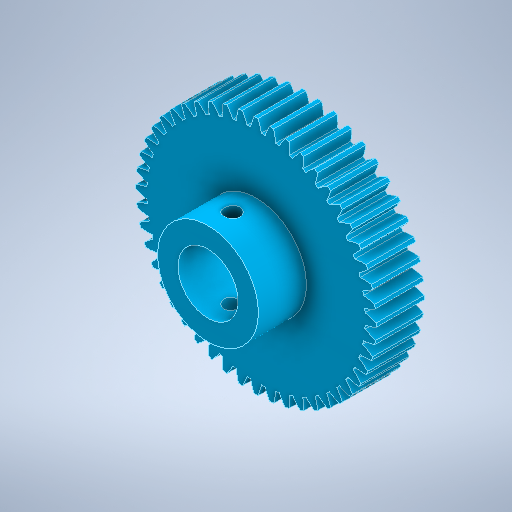
# Autodesk Inventor part: 平歯車1
Saved by Autodesk Inventor 2025.1 (Build 291241000, 241)
## iProperties
CustomPartVersion: 1
Created: 2024-10-03
Part Number: 平歯車1
Material: Steel
Document SubType Name: Modeling
Designer: yuki0520
Categories: <?xml version="1.0" encoding="UTF-16"?> <MemberInstance><Categories><FamilyTemplate><FamilyTemplateParameter ValueType="xs:double" Id="1" ObjectReferenceKey="da_z" ObjectType="kUserParameterObject"/><FamilyTemplateParameter ValueType="xs:double" Id="2" ObjectReferenceKey="da_b" ObjectType="kUserParameterObject"/><FamilyTemplateParameter ValueType="xs:double" Id="3" ObjectReferenceKey="da_beta" ObjectType="kUserParameterObject"/><FamilyTemplateParameter ValueType="xs:double" Id="4" ObjectReferenceKey="da_da" ObjectType="kUserParameterObject"/><FamilyTemplateParameter ValueType="xs:double" Id="5" ObjectReferenceKey="da_aw" ObjectType="kUserParameterObject"/><FamilyTemplateParameter ValueType="xs:string" Id="6" ObjectReferenceKey="EAIAABAAAACIAQAAAAAAAIAAAAAAAAAA" ObjectType="83910656" SubObjectId="SurfaceGeometry"/></FamilyTemplate><ParamToTemplateMap><ParamToTemplate CategoryParameter="//CategoryParameter[@InternalName='046C89C9-8512-4d59-83FE-43B91F4F132A']" TemplateParameter="1"/><ParamToTemplate CategoryParameter="//CategoryParameter[@InternalName='2552DF32-E462-4b46-AEBF-C6C7768E72AC']" TemplateParameter="2"/><ParamToTemplate CategoryParameter="//CategoryParameter[@InternalName='C9EE641D-15FC-4fae-A226-E94C4372FDD7']" TemplateParameter="3"/><ParamToTemplate><ParamToTemplate CategoryParameter="//CategoryParameter[@InternalName='00B6519A-459B-49c7-AD84-2E56D39A5744']" ConstantValue="0.000000"/></ParamToTemplate><ParamToTemplate><ParamToTemplate CategoryParameter="//CategoryParameter[@InternalName='04B31F0E-C7A6-4894-AA32-9629BEFACF47']" ConstantValue="1.000000"/></ParamToTemplate><ParamToTemplate><ParamToTemplate CategoryParameter="//CategoryParameter[@InternalName='43CBEC2E-7847-49e7-A936-2F7889FCB2D9']" ConstantValue="0.250000"/></ParamToTemplate><ParamToTemplate><ParamToTemplate CategoryParameter="//CategoryParameter[@InternalName='B1EFC894-105D-4ebd-86BF-FA20ED196853']" ConstantValue="0.350000"/></ParamToTemplate><ParamToTemplate><ParamToTemplate CategoryParameter="//CategoryParameter[@InternalName='51175063-3D10-4879-93E8-6246FE8B403D']" ConstantValue="2060000000.000000"/></ParamToTemplate><ParamToTemplate><ParamToTemplate CategoryParameter="//CategoryParameter[@InternalName='A3A52E27-4454-46a9-B0BD-C932399B70AF']" ConstantValue="0.300000"/></ParamToTemplate><ParamToTemplate><ParamToTemplate CategoryParameter="//CategoryParameter[@InternalName='91B76062-C214-41d9-B1B9-14D2AB99603D']" ConstantValue="0.100000"/></ParamToTemplate><ParamToTemplate><ParamToTemplate CategoryParameter="//CategoryParameter[@InternalName='374E806E-8B8A-4dda-A9AA-1039D6500AD2']" ConstantValue="10.000000"/></ParamToTemplate><ParamToTemplate><ParamToTemplate CategoryParameter="//CategoryParameter[@InternalName='2D373A89-B862-43d6-8D0B-0CBF12AB9F6C']" ConstantValue="0.349066"/></ParamToTemplate><ParamToTemplate CategoryParameter="//CategoryParameter[@InternalName='37777632-D6A2-4fac-9D53-DB8ACD95C989']" TemplateParameter="4"/><ParamToTemplate CategoryParameter="//CategoryParameter[@InternalName='FD1017F1-B727-4f7e-9707-0F86F1FF9423']" TemplateParameter="5"/><ParamToTemplate><ParamToTemplate CategoryParameter="//CategoryParameter[@InternalName='9E1B4470-B2D3-4ff1-B813-535BB4CDF51A']" ConstantValue="3520000.000000"/></ParamToTemplate><ParamToTemplate><ParamToTemplate CategoryParameter="//CategoryParameter[@InternalName='F8452263-BFF6-458c-9FB1-07C4B99E95CD']" ConstantValue="11400000.000000"/></ParamToTemplate><ParamToTemplate><ParamToTemplate CategoryParameter="//CategoryParameter[@InternalName='3E3BB259-FD49-497f-8171-6EBC954A3479']" ConstantValue="2.000000"/></ParamToTemplate><ParamToTemplate CategoryParameter="//CategoryParameter[@InternalName='27C3BAF2-7550-4e4b-AE2C-0DB134B7D9B7']" TemplateParameter="6"/></ParamToTemplateMap><Category DisplayName="Gear" InternalName="DC85795E-93AB-48d5-8EEE-5A27447B64BD" Mnemonic="Gear"><CategoryParameter DisplayName="z" InternalName="046C89C9-8512-4d59-83FE-43B91F4F132A" Mnemonic="z"/><CategoryParameter DisplayName="b" InternalName="2552DF32-E462-4b46-AEBF-C6C7768E72AC" Mnemonic="b"/><CategoryParameter DisplayName="||b|" InternalName="C9EE641D-15FC-4fae-A226-E94C4372FDD7" Mnemonic="beta"/><CategoryParameter DisplayName="x" InternalName="00B6519A-459B-49c7-AD84-2E56D39A5744" Mnemonic="x"/><CategoryParameter DisplayName="a*" InternalName="04B31F0E-C7A6-4894-AA32-9629BEFACF47" Mnemonic="a"/><CategoryParameter DisplayName="c*" InternalName="43CBEC2E-7847-49e7-A936-2F7889FCB2D9" Mnemonic="c"/><CategoryParameter DisplayName="r|.f|*" InternalName="B1EFC894-105D-4ebd-86BF-FA20ED196853" Mnemonic="rf"/><CategoryParameter DisplayName="E" InternalName="51175063-3D10-4879-93E8-6246FE8B403D" Mnemonic="E"/><CategoryParameter DisplayName="||m|" InternalName="A3A52E27-4454-46a9-B0BD-C932399B70AF" Mnemonic="mi"/><Category DisplayName="SpurGear" InternalName="26C5A22E-A91E-4dfd-A3B3-23CCAFAE1764" Mnemonic="SpurGear"><CategoryParameter DisplayName="m" InternalName="91B76062-C214-41d9-B1B9-14D2AB99603D" Mnemonic="m"/><CategoryParameter DisplayName="P" InternalName="374E806E-8B8A-4dda-A9AA-1039D6500AD2" Mnemonic="PP"/><CategoryParameter DisplayName="||a|" InternalName="2D373A89-B862-43d6-8D0B-0CBF12AB9F6C" Mnemonic="alpha"/><CategoryParameter DisplayName="d|.a|" InternalName="37777632-D6A2-4fac-9D53-DB8ACD95C989" Mnemonic="da"/><CategoryParameter DisplayName="a|.w|" InternalName="FD1017F1-B727-4f7e-9707-0F86F1FF9423" Mnemonic="aw"/><CategoryParameter DisplayName="||s||.Flim|" InternalName="9E1B4470-B2D3-4ff1-B813-535BB4CDF51A" Mnemonic="sFlim"/><CategoryParameter DisplayName="||s||.Hlim|" InternalName="F8452263-BFF6-458c-9FB1-07C4B99E95CD" Mnemonic="sHlim"/><CategoryParameter DisplayName="タイプ" InternalName="3E3BB259-FD49-497f-8171-6EBC954A3479" Mnemonic="type"/><CategoryParameter DisplayName="PitchDiameter" InternalName="27C3BAF2-7550-4e4b-AE2C-0DB134B7D9B7" Mnemonic="IDS_PITCHDIAM"/></Category></Category></Categories></MemberInstance>
Density: 1 g/cm^3
Appearance: スカイ ブルー 標準
Author: yuki0520
Autodesk Inventor part; units mm, degrees
sketch "Sketch1" plane through (0, 0, 0) normal (0, 0, 1) x (1, 0, 0)
  circle A0 centre (0, 0) radius 25
  dimension "d0" = 50
  constraints: 1 centre point
  measures "d0" diameter of A0
extrude "Extrusion1" add sketch "Sketch1" along normal blind 10
ref_plane "Work Plane2" through (0, 0, 5) normal (0, 0, 1) x (1, 0, 0)
sketch "Sketch2" plane through (0, 0, 0) normal (0, 0, -1) x (-1, 0, 0)
  circle A0 centre (0, 0) radius 25 projected
  circle A1 centre (0, 0) radius 24
  dimension "d3" = 48
  constraints: 1 centre point, 1 coincident
  measures "d3" diameter of A1
surface extrude "ピッチ円直径" sketch "Sketch2" against normal through all shown no curves A1
ref_plane "Work Plane8" through (0, 0, 0) normal (0.9978589, 0.0654031, 0) x (0, 0, 1)
ref_plane "Work Plane9" through (0, 0, 0) normal (1, 0, 0) x (0, 1, 0)
spur gear teeth "平歯車" teeth 48 pitch diameter 48 tip diameter 50 root diameter 45.5 face width 10 start plane through (0, 0, 0) normal (0, 0, -1) x (-1, 0, 0)
sketch "スケッチ3" plane through (0, 0, 10) normal (0, 0, 1) x (1, 0, 0)
  arc A0 (3.6683, -24.7294) -> (4.0726, -22.3825) centre (-7.7435, -21.5549) ccw projected
  arc A1 (4.0726, -22.3825) -> (4.8028, -22.2373) centre (0, 0) ccw projected
  arc A2 (4.8028, -22.2373) -> (6.0745, -24.2508) centre (15.4028, -16.9508) ccw projected
  arc A3 (6.0745, -24.2508) -> (6.8647, -24.039) centre (0, 0) ccw projected
  arc A4 (6.8647, -24.039) -> (6.9593, -21.6594) centre (-4.8638, -22.3812) ccw projected
  arc A5 (6.9593, -21.6594) -> (7.6642, -21.4201) centre (0, 0) ccw projected
  arc A6 (7.6642, -21.4201) -> (9.1879, -23.2504) centre (17.4835, -14.7953) ccw projected
  arc A7 (9.1879, -23.2504) -> (9.9437, -22.9374) centre (0, 0) ccw projected
  arc A8 (9.9437, -22.9374) -> (9.7269, -20.5658) centre (-1.9009, -22.8246) ccw projected
  arc A9 (9.7269, -20.5658) -> (10.3946, -20.2365) centre (0, 0) ccw projected
  arc A10 (10.3946, -20.2365) -> (12.1441, -21.8523) centre (19.2651, -12.3867) ccw projected
  arc A11 (12.1441, -21.8523) -> (12.8526, -21.4432) centre (0, 0) ccw projected
  arc A12 (12.8526, -21.4432) -> (12.328, -19.1202) centre (1.0946, -22.8774) ccw projected
  arc A13 (12.328, -19.1202) -> (12.947, -18.7066) centre (0, 0) ccw projected
  arc A14 (12.947, -18.7066) -> (14.8925, -20.0802) centre (20.7171, -9.7661) ccw projected
  arc A15 (14.8925, -20.0802) -> (15.5415, -19.5822) centre (0, 0) ccw projected
  arc A16 (15.5415, -19.5822) -> (14.7183, -17.3475) centre (4.0714, -22.5388) ccw projected
  arc A17 (14.7183, -17.3475) -> (15.278, -16.8566) centre (0, 0) ccw projected
  arc A18 (15.278, -16.8566) -> (17.3861, -17.9645) centre (21.8146, -6.9784) ccw projected
  arc A19 (17.3861, -17.9645) -> (17.9645, -17.3861) centre (0, 0) ccw projected
  arc A20 (17.9645, -17.3861) -> (16.8566, -15.278) centre (6.9784, -21.8146) ccw projected
  arc A21 (16.8566, -15.278) -> (17.3475, -14.7183) centre (0, 0) ccw projected
  arc A22 (17.3475, -14.7183) -> (19.5822, -15.5415) centre (22.5388, -4.0714) ccw projected
  arc A23 (19.5822, -15.5415) -> (20.0802, -14.8925) centre (0, 0) ccw projected
  arc A24 (20.0802, -14.8925) -> (18.7066, -12.947) centre (9.7661, -20.7171) ccw projected
  arc A25 (18.7066, -12.947) -> (19.1202, -12.328) centre (0, 0) ccw projected
  arc A26 (19.1202, -12.328) -> (21.4432, -12.8526) centre (22.8774, -1.0946) ccw projected
  arc A27 (21.4432, -12.8526) -> (21.8523, -12.1441) centre (0, 0) ccw projected
  arc A28 (21.8523, -12.1441) -> (20.2365, -10.3946) centre (12.3867, -19.2651) ccw projected
  arc A29 (20.2365, -10.3946) -> (20.5658, -9.7269) centre (0, 0) ccw projected
  arc A30 (20.5658, -9.7269) -> (22.9374, -9.9437) centre (22.8246, 1.9009) ccw projected
  arc A31 (22.9374, -9.9437) -> (23.2504, -9.1879) centre (0, 0) ccw projected
  arc A32 (23.2504, -9.1879) -> (21.4201, -7.6642) centre (14.7953, -17.4835) ccw projected
  arc A33 (21.4201, -7.6642) -> (21.6594, -6.9593) centre (0, 0) ccw projected
  arc A34 (21.6594, -6.9593) -> (24.039, -6.8647) centre (22.3812, 4.8638) ccw projected
  arc A35 (24.039, -6.8647) -> (24.2508, -6.0745) centre (0, 0) ccw projected
  arc A36 (24.2508, -6.0745) -> (22.2373, -4.8028) centre (16.9508, -15.4028) ccw projected
  arc A37 (22.2373, -4.8028) -> (22.3825, -4.0726) centre (0, 0) ccw projected
  arc A38 (22.3825, -4.0726) -> (24.7294, -3.6683) centre (21.5549, 7.7435) ccw projected
  arc A39 (24.7294, -3.6683) -> (24.8362, -2.8572) centre (0, 0) ccw projected
  arc A40 (24.8362, -2.8572) -> (22.6739, -1.8592) centre (18.8162, -13.0585) ccw projected
  arc A41 (22.6739, -1.8592) -> (22.7226, -1.1163) centre (0, 0) ccw projected
  arc A42 (22.7226, -1.1163) -> (24.9967, -0.409) centre (20.3597, 10.4907) ccw projected
  arc A43 (24.9967, -0.409) -> (24.9967, 0.409) centre (0, 0) ccw projected
  arc A44 (24.9967, 0.409) -> (22.7226, 1.1163) centre (20.3597, -10.4907) ccw projected
  arc A45 (22.7226, 1.1163) -> (22.6739, 1.8592) centre (0, 0) ccw projected
  arc A46 (22.6739, 1.8592) -> (24.8362, 2.8572) centre (18.8162, 13.0585) ccw projected
  arc A47 (24.8362, 2.8572) -> (24.7294, 3.6683) centre (0, 0) ccw projected
  arc A48 (24.7294, 3.6683) -> (22.3825, 4.0726) centre (21.5549, -7.7435) ccw projected
  arc A49 (22.3825, 4.0726) -> (22.2373, 4.8028) centre (0, 0) ccw projected
  arc A50 (22.2373, 4.8028) -> (24.2508, 6.0745) centre (16.9508, 15.4028) ccw projected
  arc A51 (24.2508, 6.0745) -> (24.039, 6.8647) centre (0, 0) ccw projected
  arc A52 (24.039, 6.8647) -> (21.6594, 6.9593) centre (22.3812, -4.8638) ccw projected
  arc A53 (21.6594, 6.9593) -> (21.4201, 7.6642) centre (0, 0) ccw projected
  arc A54 (21.4201, 7.6642) -> (23.2504, 9.1879) centre (14.7953, 17.4835) ccw projected
  arc A55 (23.2504, 9.1879) -> (22.9374, 9.9437) centre (0, 0) ccw projected
  arc A56 (22.9374, 9.9437) -> (20.5658, 9.7269) centre (22.8246, -1.9009) ccw projected
  arc A57 (20.5658, 9.7269) -> (20.2365, 10.3946) centre (0, 0) ccw projected
  arc A58 (20.2365, 10.3946) -> (21.8523, 12.1441) centre (12.3867, 19.2651) ccw projected
  arc A59 (21.8523, 12.1441) -> (21.4432, 12.8526) centre (0, 0) ccw projected
  arc A60 (21.4432, 12.8526) -> (19.1202, 12.328) centre (22.8774, 1.0946) ccw projected
  arc A61 (19.1202, 12.328) -> (18.7066, 12.947) centre (0, 0) ccw projected
  arc A62 (18.7066, 12.947) -> (20.0802, 14.8925) centre (9.7661, 20.7171) ccw projected
  arc A63 (20.0802, 14.8925) -> (19.5822, 15.5415) centre (0, 0) ccw projected
  arc A64 (19.5822, 15.5415) -> (17.3475, 14.7183) centre (22.5388, 4.0714) ccw projected
  arc A65 (17.3475, 14.7183) -> (16.8566, 15.278) centre (0, 0) ccw projected
  arc A66 (16.8566, 15.278) -> (17.9645, 17.3861) centre (6.9784, 21.8146) ccw projected
  arc A67 (17.9645, 17.3861) -> (17.3861, 17.9645) centre (0, 0) ccw projected
  arc A68 (17.3861, 17.9645) -> (15.278, 16.8566) centre (21.8146, 6.9784) ccw projected
  arc A69 (15.278, 16.8566) -> (14.7183, 17.3475) centre (0, 0) ccw projected
  arc A70 (14.7183, 17.3475) -> (15.5415, 19.5822) centre (4.0714, 22.5388) ccw projected
  arc A71 (15.5415, 19.5822) -> (14.8925, 20.0802) centre (0, 0) ccw projected
  arc A72 (14.8925, 20.0802) -> (12.947, 18.7066) centre (20.7171, 9.7661) ccw projected
  arc A73 (12.947, 18.7066) -> (12.328, 19.1202) centre (0, 0) ccw projected
  arc A74 (12.328, 19.1202) -> (12.8526, 21.4432) centre (1.0946, 22.8774) ccw projected
  arc A75 (12.8526, 21.4432) -> (12.1441, 21.8523) centre (0, 0) ccw projected
  arc A76 (12.1441, 21.8523) -> (10.3946, 20.2365) centre (19.2651, 12.3867) ccw projected
  arc A77 (10.3946, 20.2365) -> (9.7269, 20.5658) centre (0, 0) ccw projected
  arc A78 (9.7269, 20.5658) -> (9.9437, 22.9374) centre (-1.9009, 22.8246) ccw projected
  arc A79 (9.9437, 22.9374) -> (9.1879, 23.2504) centre (0, 0) ccw projected
  arc A80 (9.1879, 23.2504) -> (7.6642, 21.4201) centre (17.4835, 14.7953) ccw projected
  arc A81 (7.6642, 21.4201) -> (6.9593, 21.6594) centre (0, 0) ccw projected
  arc A82 (6.9593, 21.6594) -> (6.8647, 24.039) centre (-4.8638, 22.3812) ccw projected
  arc A83 (6.8647, 24.039) -> (6.0745, 24.2508) centre (0, 0) ccw projected
  arc A84 (6.0745, 24.2508) -> (4.8028, 22.2373) centre (15.4028, 16.9508) ccw projected
  arc A85 (4.8028, 22.2373) -> (4.0726, 22.3825) centre (0, 0) ccw projected
  arc A86 (4.0726, 22.3825) -> (3.6683, 24.7294) centre (-7.7435, 21.5549) ccw projected
  arc A87 (3.6683, 24.7294) -> (2.8572, 24.8362) centre (0, 0) ccw projected
  arc A88 (2.8572, 24.8362) -> (1.8592, 22.6739) centre (13.0585, 18.8162) ccw projected
  arc A89 (1.8592, 22.6739) -> (1.1163, 22.7226) centre (0, 0) ccw projected
  arc A90 (1.1163, 22.7226) -> (0.409, 24.9967) centre (-10.4907, 20.3597) ccw projected
  arc A91 (0.409, 24.9967) -> (-0.409, 24.9967) centre (0, 0) ccw projected
  arc A92 (-0.409, 24.9967) -> (-1.1163, 22.7226) centre (10.4907, 20.3597) ccw projected
  arc A93 (-1.1163, 22.7226) -> (-1.8592, 22.6739) centre (0, 0) ccw projected
  arc A94 (-1.8592, 22.6739) -> (-2.8572, 24.8362) centre (-13.0585, 18.8162) ccw projected
  arc A95 (2.8572, -24.8362) -> (3.6683, -24.7294) centre (0, 0) ccw projected
  circle A96 centre (0, 0) radius 22.75
  arc A97 (-3.6683, 24.7294) -> (-4.0726, 22.3825) centre (7.7435, 21.5549) ccw projected
  arc A98 (-4.0726, 22.3825) -> (-4.8028, 22.2373) centre (0, 0) ccw projected
  arc A99 (-4.8028, 22.2373) -> (-6.0745, 24.2508) centre (-15.4028, 16.9508) ccw projected
  arc A100 (-6.0745, 24.2508) -> (-6.8647, 24.039) centre (0, 0) ccw projected
  arc A101 (-6.8647, 24.039) -> (-6.9593, 21.6594) centre (4.8638, 22.3812) ccw projected
  arc A102 (-6.9593, 21.6594) -> (-7.6642, 21.4201) centre (0, 0) ccw projected
  arc A103 (-7.6642, 21.4201) -> (-9.1879, 23.2504) centre (-17.4835, 14.7953) ccw projected
  arc A104 (-9.1879, 23.2504) -> (-9.9437, 22.9374) centre (0, 0) ccw projected
  arc A105 (-9.9437, 22.9374) -> (-9.7269, 20.5658) centre (1.9009, 22.8246) ccw projected
  arc A106 (-9.7269, 20.5658) -> (-10.3946, 20.2365) centre (0, 0) ccw projected
  arc A107 (-10.3946, 20.2365) -> (-12.1441, 21.8523) centre (-19.2651, 12.3867) ccw projected
  arc A108 (-12.1441, 21.8523) -> (-12.8526, 21.4432) centre (0, 0) ccw projected
  arc A109 (-12.8526, 21.4432) -> (-12.328, 19.1202) centre (-1.0946, 22.8774) ccw projected
  arc A110 (-12.328, 19.1202) -> (-12.947, 18.7066) centre (0, 0) ccw projected
  arc A111 (-12.947, 18.7066) -> (-14.8925, 20.0802) centre (-20.7171, 9.7661) ccw projected
  arc A112 (-14.8925, 20.0802) -> (-15.5415, 19.5822) centre (0, 0) ccw projected
  arc A113 (-15.5415, 19.5822) -> (-14.7183, 17.3475) centre (-4.0714, 22.5388) ccw projected
  arc A114 (-14.7183, 17.3475) -> (-15.278, 16.8566) centre (0, 0) ccw projected
  arc A115 (-15.278, 16.8566) -> (-17.3861, 17.9645) centre (-21.8146, 6.9784) ccw projected
  arc A116 (-17.3861, 17.9645) -> (-17.9645, 17.3861) centre (0, 0) ccw projected
  arc A117 (-17.9645, 17.3861) -> (-16.8566, 15.278) centre (-6.9784, 21.8146) ccw projected
  arc A118 (-16.8566, 15.278) -> (-17.3475, 14.7183) centre (0, 0) ccw projected
  arc A119 (-17.3475, 14.7183) -> (-19.5822, 15.5415) centre (-22.5388, 4.0714) ccw projected
  arc A120 (-19.5822, 15.5415) -> (-20.0802, 14.8925) centre (0, 0) ccw projected
  arc A121 (-20.0802, 14.8925) -> (-18.7066, 12.947) centre (-9.7661, 20.7171) ccw projected
  arc A122 (-18.7066, 12.947) -> (-19.1202, 12.328) centre (0, 0) ccw projected
  arc A123 (-19.1202, 12.328) -> (-21.4432, 12.8526) centre (-22.8774, 1.0946) ccw projected
  arc A124 (-21.4432, 12.8526) -> (-21.8523, 12.1441) centre (0, 0) ccw projected
  arc A125 (-21.8523, 12.1441) -> (-20.2365, 10.3946) centre (-12.3867, 19.2651) ccw projected
  arc A126 (-20.2365, 10.3946) -> (-20.5658, 9.7269) centre (0, 0) ccw projected
  arc A127 (-20.5658, 9.7269) -> (-22.9374, 9.9437) centre (-22.8246, -1.9009) ccw projected
  arc A128 (-22.9374, 9.9437) -> (-23.2504, 9.1879) centre (0, 0) ccw projected
  arc A129 (-23.2504, 9.1879) -> (-21.4201, 7.6642) centre (-14.7953, 17.4835) ccw projected
  arc A130 (-21.4201, 7.6642) -> (-21.6594, 6.9593) centre (0, 0) ccw projected
  arc A131 (-21.6594, 6.9593) -> (-24.039, 6.8647) centre (-22.3812, -4.8638) ccw projected
  arc A132 (-24.039, 6.8647) -> (-24.2508, 6.0745) centre (0, 0) ccw projected
  arc A133 (-24.2508, 6.0745) -> (-22.2373, 4.8028) centre (-16.9508, 15.4028) ccw projected
  arc A134 (-22.2373, 4.8028) -> (-22.3825, 4.0726) centre (0, 0) ccw projected
  arc A135 (-22.3825, 4.0726) -> (-24.7294, 3.6683) centre (-21.5549, -7.7435) ccw projected
  arc A136 (-24.7294, 3.6683) -> (-24.8362, 2.8572) centre (0, 0) ccw projected
  arc A137 (-24.8362, 2.8572) -> (-22.6739, 1.8592) centre (-18.8162, 13.0585) ccw projected
  arc A138 (-22.6739, 1.8592) -> (-22.7226, 1.1163) centre (0, 0) ccw projected
  arc A139 (-22.7226, 1.1163) -> (-24.9967, 0.409) centre (-20.3597, -10.4907) ccw projected
  arc A140 (-24.9967, 0.409) -> (-24.9967, -0.409) centre (0, 0) ccw projected
  arc A141 (-24.9967, -0.409) -> (-22.7226, -1.1163) centre (-20.3597, 10.4907) ccw projected
  arc A142 (-22.7226, -1.1163) -> (-22.6739, -1.8592) centre (0, 0) ccw projected
  arc A143 (-22.6739, -1.8592) -> (-24.8362, -2.8572) centre (-18.8162, -13.0585) ccw projected
  arc A144 (-24.8362, -2.8572) -> (-24.7294, -3.6683) centre (0, 0) ccw projected
  arc A145 (-24.7294, -3.6683) -> (-22.3825, -4.0726) centre (-21.5549, 7.7435) ccw projected
  arc A146 (-22.3825, -4.0726) -> (-22.2373, -4.8028) centre (0, 0) ccw projected
  arc A147 (-22.2373, -4.8028) -> (-24.2508, -6.0745) centre (-16.9508, -15.4028) ccw projected
  arc A148 (-24.2508, -6.0745) -> (-24.039, -6.8647) centre (0, 0) ccw projected
  arc A149 (-24.039, -6.8647) -> (-21.6594, -6.9593) centre (-22.3812, 4.8638) ccw projected
  arc A150 (-21.6594, -6.9593) -> (-21.4201, -7.6642) centre (0, 0) ccw projected
  arc A151 (-21.4201, -7.6642) -> (-23.2504, -9.1879) centre (-14.7953, -17.4835) ccw projected
  arc A152 (-23.2504, -9.1879) -> (-22.9374, -9.9437) centre (0, 0) ccw projected
  arc A153 (-22.9374, -9.9437) -> (-20.5658, -9.7269) centre (-22.8246, 1.9009) ccw projected
  arc A154 (-20.5658, -9.7269) -> (-20.2365, -10.3946) centre (0, 0) ccw projected
  arc A155 (-20.2365, -10.3946) -> (-21.8523, -12.1441) centre (-12.3867, -19.2651) ccw projected
  arc A156 (-21.8523, -12.1441) -> (-21.4432, -12.8526) centre (0, 0) ccw projected
  arc A157 (-21.4432, -12.8526) -> (-19.1202, -12.328) centre (-22.8774, -1.0946) ccw projected
  arc A158 (-19.1202, -12.328) -> (-18.7066, -12.947) centre (0, 0) ccw projected
  arc A159 (-18.7066, -12.947) -> (-20.0802, -14.8925) centre (-9.7661, -20.7171) ccw projected
  arc A160 (-20.0802, -14.8925) -> (-19.5822, -15.5415) centre (0, 0) ccw projected
  arc A161 (-19.5822, -15.5415) -> (-17.3475, -14.7183) centre (-22.5388, -4.0714) ccw projected
  arc A162 (-17.3475, -14.7183) -> (-16.8566, -15.278) centre (0, 0) ccw projected
  arc A163 (-16.8566, -15.278) -> (-17.9645, -17.3861) centre (-6.9784, -21.8146) ccw projected
  arc A164 (-17.9645, -17.3861) -> (-17.3861, -17.9645) centre (0, 0) ccw projected
  arc A165 (-17.3861, -17.9645) -> (-15.278, -16.8566) centre (-21.8146, -6.9784) ccw projected
  arc A166 (-15.278, -16.8566) -> (-14.7183, -17.3475) centre (0, 0) ccw projected
  arc A167 (-14.7183, -17.3475) -> (-15.5415, -19.5822) centre (-4.0714, -22.5388) ccw projected
  arc A168 (-15.5415, -19.5822) -> (-14.8925, -20.0802) centre (0, 0) ccw projected
  arc A169 (-14.8925, -20.0802) -> (-12.947, -18.7066) centre (-20.7171, -9.7661) ccw projected
  arc A170 (-12.947, -18.7066) -> (-12.328, -19.1202) centre (0, 0) ccw projected
  arc A171 (-12.328, -19.1202) -> (-12.8526, -21.4432) centre (-1.0946, -22.8774) ccw projected
  arc A172 (-12.8526, -21.4432) -> (-12.1441, -21.8523) centre (0, 0) ccw projected
  arc A173 (-12.1441, -21.8523) -> (-10.3946, -20.2365) centre (-19.2651, -12.3867) ccw projected
  arc A174 (-10.3946, -20.2365) -> (-9.7269, -20.5658) centre (0, 0) ccw projected
  arc A175 (-9.7269, -20.5658) -> (-9.9437, -22.9374) centre (1.9009, -22.8246) ccw projected
  arc A176 (-9.9437, -22.9374) -> (-9.1879, -23.2504) centre (0, 0) ccw projected
  arc A177 (-9.1879, -23.2504) -> (-7.6642, -21.4201) centre (-17.4835, -14.7953) ccw projected
  arc A178 (-7.6642, -21.4201) -> (-6.9593, -21.6594) centre (0, 0) ccw projected
  arc A179 (-6.9593, -21.6594) -> (-6.8647, -24.039) centre (4.8638, -22.3812) ccw projected
  arc A180 (-6.8647, -24.039) -> (-6.0745, -24.2508) centre (0, 0) ccw projected
  arc A181 (-6.0745, -24.2508) -> (-4.8028, -22.2373) centre (-15.4028, -16.9508) ccw projected
  arc A182 (-4.8028, -22.2373) -> (-4.0726, -22.3825) centre (0, 0) ccw projected
  arc A183 (-4.0726, -22.3825) -> (-3.6683, -24.7294) centre (7.7435, -21.5549) ccw projected
  arc A184 (-3.6683, -24.7294) -> (-2.8572, -24.8362) centre (0, 0) ccw projected
  arc A185 (-2.8572, -24.8362) -> (-1.8592, -22.6739) centre (-13.0585, -18.8162) ccw projected
  arc A186 (-1.8592, -22.6739) -> (-1.1163, -22.7226) centre (0, 0) ccw projected
  arc A187 (-1.1163, -22.7226) -> (-0.409, -24.9967) centre (10.4907, -20.3597) ccw projected
  arc A188 (-0.409, -24.9967) -> (0.409, -24.9967) centre (0, 0) ccw projected
  arc A189 (0.409, -24.9967) -> (1.1163, -22.7226) centre (-10.4907, -20.3597) ccw projected
  arc A190 (1.1163, -22.7226) -> (1.8592, -22.6739) centre (0, 0) ccw projected
  arc A191 (1.8592, -22.6739) -> (2.8572, -24.8362) centre (13.0585, -18.8162) ccw projected
  arc A192 (-2.8572, 24.8362) -> (-3.6683, 24.7294) centre (0, 0) ccw projected
  circle A193 centre (0, 0) radius 10.5
  point P0 (15.278, -16.8566)
  point P1 (16.8566, -15.278)
  point P2 (17.3475, -14.7183)
  point P3 (18.7066, -12.947)
  point P4 (19.1202, -12.328)
  point P5 (20.2365, -10.3946)
  point P6 (20.5658, -9.7269)
  point P7 (21.4201, -7.6642)
  point P8 (21.6594, -6.9593)
  point P9 (22.2373, -4.8028)
  point P10 (22.3825, -4.0726)
  point P11 (22.6739, -1.8592)
  point P12 (22.7226, -1.1163)
  point P13 (22.7226, 1.1163)
  point P14 (22.6739, 1.8592)
  point P15 (21.6594, 6.9593)
  point P16 (21.4201, 7.6642)
  point P17 (20.5658, 9.7269)
  point P18 (20.2365, 10.3946)
  point P19 (19.1202, 12.328)
  point P20 (18.7066, 12.947)
  point P21 (17.3475, 14.7183)
  point P22 (16.8566, 15.278)
  point P23 (15.278, 16.8566)
  point P24 (14.7183, 17.3475)
  point P25 (12.947, 18.7066)
  point P26 (10.3946, 20.2365)
  point P27 (9.7269, 20.5658)
  point P28 (7.6642, 21.4201)
  point P29 (4.8028, 22.2373)
  point P30 (4.0726, 22.3825)
  point P31 (1.8592, 22.6739)
  point P32 (1.1163, 22.7226)
  point P33 (-1.8592, 22.6739)
  point P34 (4.0726, -22.3825)
  point P35 (4.8028, -22.2373)
  point P36 (6.9593, -21.6594)
  point P37 (7.6642, -21.4201)
  point P38 (9.7269, -20.5658)
  point P39 (10.3946, -20.2365)
  point P40 (12.328, -19.1202)
  point P41 (12.947, -18.7066)
  point P42 (14.7183, -17.3475)
  dimension "d63" = 21
  constraints: 2 coincident, 1 centre point, 3 other
  measures "d63" diameter of A193
extrude "押し出し2" add sketch "スケッチ3" along normal blind 10 contours A193
sketch "スケッチ4" plane through (0, 0, 0) normal (0, 0, -1) x (-1, 0, 0)
  circle A0 centre (0, 0) radius 6.25
  dimension "d51" = 12.5
  constraints: 1 centre point, 1 coincident
  measures "d51" diameter of A0
extrude "押し出し3" cut sketch "スケッチ4" against normal blind 100
sketch "スケッチ6" plane through (0, 0, 0) normal (0, 1, 0) x (-1, 0, 0)
  line L0 (10.5, 20) -> (-10.5, 20) projected
  line L1 (-10.5, 10) -> (10.5, 10) projected
  line L2 (0, 20) -> (0, 0)
  line L3 (6.25, 0) -> (-6.25, 0) projected
  line L4 (4.0726, 0) -> (3.6683, 0) projected
  line L5 (3.6683, 0) -> (2.8572, 0) projected
  line L6 (2.8572, 0) -> (1.8592, 0) projected
  line L7 (1.8592, 0) -> (1.1163, 0) projected
  line L8 (1.1163, 0) -> (0.409, 0) projected
  line L9 (0.409, 0) -> (-0.409, 0) projected
  line L10 (-0.409, 0) -> (-1.1163, 0) projected
  line L11 (-1.1163, 0) -> (-1.8592, 0) projected
  line L12 (-1.8592, 0) -> (-2.8572, 0) projected
  line L13 (-2.8572, 0) -> (-3.6683, 0) projected
  line L14 (-3.6683, 0) -> (-4.0726, 0) projected
  line L15 (-4.0726, 0) -> (-4.8028, 0) projected
  line L16 (-4.8028, 0) -> (-6.0745, 0) projected
  line L17 (-6.0745, 0) -> (-6.8647, 0) projected
  line L18 (-6.8647, 0) -> (-6.9593, 0) projected
  line L19 (-6.9593, 0) -> (-7.6642, 0) projected
  line L20 (-7.6642, 0) -> (-9.1879, 0) projected
  line L21 (-9.1879, 0) -> (-9.9437, 0) projected
  line L22 (-9.9437, 0) -> (-9.7269, 0) projected
  line L23 (-9.7269, 0) -> (-10.3946, 0) projected
  line L24 (-10.3946, 0) -> (-12.1441, 0) projected
  line L25 (-12.1441, 0) -> (-12.8526, 0) projected
  line L26 (-12.8526, 0) -> (-12.328, 0) projected
  line L27 (-12.328, 0) -> (-12.947, 0) projected
  line L28 (-12.947, 0) -> (-14.8925, 0) projected
  line L29 (-14.8925, 0) -> (-15.5415, 0) projected
  line L30 (-15.5415, 0) -> (-14.7183, 0) projected
  line L31 (-14.7183, 0) -> (-15.278, 0) projected
  line L32 (-15.278, 0) -> (-17.3861, 0) projected
  line L33 (-17.3861, 0) -> (-17.9645, 0) projected
  line L34 (-17.9645, 0) -> (-16.8566, 0) projected
  line L35 (-16.8566, 0) -> (-17.3475, 0) projected
  line L36 (-17.3475, 0) -> (-19.5822, 0) projected
  line L37 (-19.5822, 0) -> (-20.0802, 0) projected
  line L38 (-20.0802, 0) -> (-18.7066, 0) projected
  line L39 (-18.7066, 0) -> (-19.1202, 0) projected
  line L40 (-19.1202, 0) -> (-21.4432, 0) projected
  line L41 (-21.4432, 0) -> (-21.8523, 0) projected
  line L42 (-21.8523, 0) -> (-20.2365, 0) projected
  line L43 (-20.2365, 0) -> (-20.5658, 0) projected
  line L44 (-20.5658, 0) -> (-22.9374, 0) projected
  line L45 (-22.9374, 0) -> (-23.2504, 0) projected
  line L46 (-23.2504, 0) -> (-21.4201, 0) projected
  line L47 (-21.4201, 0) -> (-21.6594, 0) projected
  line L48 (-21.6594, 0) -> (-24.039, 0) projected
  line L49 (-24.039, 0) -> (-24.2508, 0) projected
  line L50 (-24.2508, 0) -> (-22.2373, 0) projected
  line L51 (-22.2373, 0) -> (-22.3825, 0) projected
  line L52 (-22.3825, 0) -> (-24.7294, 0) projected
  line L53 (-24.7294, 0) -> (-24.8362, 0) projected
  line L54 (-24.8362, 0) -> (-22.6739, 0) projected
  line L55 (-22.6739, 0) -> (-22.7226, 0) projected
  line L56 (-22.7226, 0) -> (-24.9967, 0) projected
  line L57 (-24.9967, 0) -> (-24.9967, 0) projected
  line L58 (-24.9967, 0) -> (-22.7226, 0) projected
  line L59 (-22.7226, 0) -> (-22.6739, 0) projected
  line L60 (-22.6739, 0) -> (-24.8362, 0) projected
  line L61 (-24.8362, 0) -> (-24.7294, 0) projected
  line L62 (-24.7294, 0) -> (-22.3825, 0) projected
  line L63 (-22.3825, 0) -> (-22.2373, 0) projected
  line L64 (-22.2373, 0) -> (-24.2508, 0) projected
  line L65 (-24.2508, 0) -> (-24.039, 0) projected
  line L66 (-24.039, 0) -> (-21.6594, 0) projected
  line L67 (-21.6594, 0) -> (-21.4201, 0) projected
  line L68 (-21.4201, 0) -> (-23.2504, 0) projected
  line L69 (-23.2504, 0) -> (-22.9374, 0) projected
  line L70 (-22.9374, 0) -> (-20.5658, 0) projected
  line L71 (-20.5658, 0) -> (-20.2365, 0) projected
  line L72 (-20.2365, 0) -> (-21.8523, 0) projected
  line L73 (-21.8523, 0) -> (-21.4432, 0) projected
  line L74 (-21.4432, 0) -> (-19.1202, 0) projected
  line L75 (-19.1202, 0) -> (-18.7066, 0) projected
  line L76 (-18.7066, 0) -> (-20.0802, 0) projected
  line L77 (-20.0802, 0) -> (-19.5822, 0) projected
  line L78 (-19.5822, 0) -> (-17.3475, 0) projected
  line L79 (-17.3475, 0) -> (-16.8566, 0) projected
  line L80 (-16.8566, 0) -> (-17.9645, 0) projected
  line L81 (-17.9645, 0) -> (-17.3861, 0) projected
  line L82 (-17.3861, 0) -> (-15.278, 0) projected
  line L83 (-15.278, 0) -> (-14.7183, 0) projected
  line L84 (-14.7183, 0) -> (-15.5415, 0) projected
  line L85 (-15.5415, 0) -> (-14.8925, 0) projected
  line L86 (-14.8925, 0) -> (-12.947, 0) projected
  line L87 (-12.947, 0) -> (-12.328, 0) projected
  line L88 (-12.328, 0) -> (-12.8526, 0) projected
  line L89 (-12.8526, 0) -> (-12.1441, 0) projected
  line L90 (-12.1441, 0) -> (-10.3946, 0) projected
  line L91 (-10.3946, 0) -> (-9.7269, 0) projected
  line L92 (-9.7269, 0) -> (-9.9437, 0) projected
  line L93 (-9.9437, 0) -> (-9.1879, 0) projected
  line L94 (-9.1879, 0) -> (-7.6642, 0) projected
  line L95 (-7.6642, 0) -> (-6.9593, 0) projected
  line L96 (-6.9593, 0) -> (-6.8647, 0) projected
  line L97 (-6.8647, 0) -> (-6.0745, 0) projected
  line L98 (-6.0745, 0) -> (-4.8028, 0) projected
  line L99 (-4.8028, 0) -> (-4.0726, 0) projected
  line L100 (-4.0726, 0) -> (-3.6683, 0) projected
  line L101 (-3.6683, 0) -> (-2.8572, 0) projected
  line L102 (-2.8572, 0) -> (-1.8592, 0) projected
  line L103 (-1.8592, 0) -> (-1.1163, 0) projected
  line L104 (-1.1163, 0) -> (-0.409, 0) projected
  line L105 (-0.409, 0) -> (0.409, 0) projected
  line L106 (0.409, 0) -> (1.1163, 0) projected
  line L107 (1.1163, 0) -> (1.8592, 0) projected
  line L108 (1.8592, 0) -> (2.8572, 0) projected
  line L109 (2.8572, 0) -> (3.6683, 0) projected
  line L110 (3.6683, 0) -> (4.0726, 0) projected
  line L111 (4.0726, 0) -> (4.8028, 0) projected
  line L112 (4.8028, 0) -> (6.0745, 0) projected
  line L113 (6.0745, 0) -> (6.8647, 0) projected
  line L114 (6.8647, 0) -> (6.9593, 0) projected
  line L115 (6.9593, 0) -> (7.6642, 0) projected
  line L116 (7.6642, 0) -> (9.1879, 0) projected
  line L117 (9.1879, 0) -> (9.9437, 0) projected
  line L118 (9.9437, 0) -> (9.7269, 0) projected
  line L119 (9.7269, 0) -> (10.3946, 0) projected
  line L120 (10.3946, 0) -> (12.1441, 0) projected
  line L121 (12.1441, 0) -> (12.8526, 0) projected
  line L122 (12.8526, 0) -> (12.328, 0) projected
  line L123 (12.328, 0) -> (12.947, 0) projected
  line L124 (12.947, 0) -> (14.8925, 0) projected
  line L125 (14.8925, 0) -> (15.5415, 0) projected
  line L126 (15.5415, 0) -> (14.7183, 0) projected
  line L127 (14.7183, 0) -> (15.278, 0) projected
  line L128 (15.278, 0) -> (17.3861, 0) projected
  line L129 (17.3861, 0) -> (17.9645, 0) projected
  line L130 (17.9645, 0) -> (16.8566, 0) projected
  line L131 (16.8566, 0) -> (17.3475, 0) projected
  line L132 (17.3475, 0) -> (19.5822, 0) projected
  line L133 (19.5822, 0) -> (20.0802, 0) projected
  line L134 (20.0802, 0) -> (18.7066, 0) projected
  line L135 (18.7066, 0) -> (19.1202, 0) projected
  line L136 (19.1202, 0) -> (21.4432, 0) projected
  line L137 (21.4432, 0) -> (21.8523, 0) projected
  line L138 (21.8523, 0) -> (20.2365, 0) projected
  line L139 (20.2365, 0) -> (20.5658, 0) projected
  line L140 (20.5658, 0) -> (22.9374, 0) projected
  line L141 (22.9374, 0) -> (23.2504, 0) projected
  line L142 (23.2504, 0) -> (21.4201, 0) projected
  line L143 (21.4201, 0) -> (21.6594, 0) projected
  line L144 (21.6594, 0) -> (24.039, 0) projected
  line L145 (24.039, 0) -> (24.2508, 0) projected
  line L146 (24.2508, 0) -> (22.2373, 0) projected
  line L147 (22.2373, 0) -> (22.3825, 0) projected
  line L148 (22.3825, 0) -> (24.7294, 0) projected
  line L149 (24.7294, 0) -> (24.8362, 0) projected
  line L150 (24.8362, 0) -> (22.6739, 0) projected
  line L151 (22.6739, 0) -> (22.7226, 0) projected
  line L152 (22.7226, 0) -> (24.9967, 0) projected
  line L153 (24.9967, 0) -> (24.9967, 0) projected
  line L154 (24.9967, 0) -> (22.7226, 0) projected
  line L155 (22.7226, 0) -> (22.6739, 0) projected
  line L156 (22.6739, 0) -> (24.8362, 0) projected
  line L157 (24.8362, 0) -> (24.7294, 0) projected
  line L158 (24.7294, 0) -> (22.3825, 0) projected
  line L159 (22.3825, 0) -> (22.2373, 0) projected
  line L160 (22.2373, 0) -> (24.2508, 0) projected
  line L161 (24.2508, 0) -> (24.039, 0) projected
  line L162 (24.039, 0) -> (21.6594, 0) projected
  line L163 (21.6594, 0) -> (21.4201, 0) projected
  line L164 (21.4201, 0) -> (23.2504, 0) projected
  line L165 (23.2504, 0) -> (22.9374, 0) projected
  line L166 (22.9374, 0) -> (20.5658, 0) projected
  line L167 (20.5658, 0) -> (20.2365, 0) projected
  line L168 (20.2365, 0) -> (21.8523, 0) projected
  line L169 (21.8523, 0) -> (21.4432, 0) projected
  line L170 (21.4432, 0) -> (19.1202, 0) projected
  line L171 (19.1202, 0) -> (18.7066, 0) projected
  line L172 (18.7066, 0) -> (20.0802, 0) projected
  line L173 (20.0802, 0) -> (19.5822, 0) projected
  line L174 (19.5822, 0) -> (17.3475, 0) projected
  line L175 (17.3475, 0) -> (16.8566, 0) projected
  line L176 (16.8566, 0) -> (17.9645, 0) projected
  line L177 (17.9645, 0) -> (17.3861, 0) projected
  line L178 (17.3861, 0) -> (15.278, 0) projected
  line L179 (15.278, 0) -> (14.7183, 0) projected
  line L180 (14.7183, 0) -> (15.5415, 0) projected
  line L181 (15.5415, 0) -> (14.8925, 0) projected
  line L182 (14.8925, 0) -> (12.947, 0) projected
  line L183 (12.947, 0) -> (12.328, 0) projected
  line L184 (12.328, 0) -> (12.8526, 0) projected
  line L185 (12.8526, 0) -> (12.1441, 0) projected
  line L186 (12.1441, 0) -> (10.3946, 0) projected
  line L187 (10.3946, 0) -> (9.7269, 0) projected
  line L188 (9.7269, 0) -> (9.9437, 0) projected
  line L189 (9.9437, 0) -> (9.1879, 0) projected
  line L190 (9.1879, 0) -> (7.6642, 0) projected
  line L191 (7.6642, 0) -> (6.9593, 0) projected
  line L192 (6.9593, 0) -> (6.8647, 0) projected
  line L193 (6.8647, 0) -> (6.0745, 0) projected
  line L194 (6.0745, 0) -> (4.8028, 0) projected
  line L195 (4.8028, 0) -> (4.0726, 0) projected
  point P0 (0, 15)
  dimension "d64" = 5
  constraints: 2 end point, 1 midpoint, 1 point on line, 1 vertical
  measures "d64" distance from line of L0 point (0, 15)
hole "穴2" at (0, 0, 15) direction (0, -1, 0) diameter 3.3 end through all both
equation "\"d0\" = da_da"
equation "\"d1\" = da_b"
equation "\"d3\" = da_d"
equation "\"d16\" = da_aw"
equation "\"d43\" = da_aw"
equation "\"d46\" = da_aw"
equation "\"da_da\" = 50"
equation "\"da_b\" = 10"
equation "\"da_d\" = 48"
equation "\"da_aw\" = 48"
body "Solid1"
body "Srf1"
